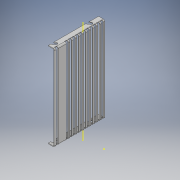
# Autodesk Inventor part: Einschub
Saved by Autodesk Inventor 2018 (Build 220112000, 112)
## iProperties
Created: 2017-11-15
Part Number: Einschub
Material: Generisch
Document SubType Name: Blech
Designer: aXe
Density: 1 g/cm^3
Sheet Metal Rule: Standard_mm
Appearance: Vorgabe
Flat Pattern Width: 14.3 cm
Flat Pattern Length: 27.2048 cm
Flat Pattern Area: 389.028 cm^2
Sheet Metal Width: 143,000 mm
Sheet Metal Length: 272,048 mm
Sheet Metal Area: 38902,834 mm^2
Author: aXe
Autodesk Inventor part; units mm, degrees
ref_plane "YZ Plane" through (0, 0, 0) normal (1, 0, 0) x (0, 1, 0)
ref_plane "XZ Plane" through (0, 0, 0) normal (0, 1, 0) x (-1, 0, 0)
ref_plane "XY Plane" through (0, 0, 0) normal (0, 0, 1) x (1, 0, 0)
ref_plane "Arbeitsebene1" through (-78, 16.4731, 8) normal (1, 0, 0) x (0, 0, 1)
sketch "Skizze1" plane through (-78, 16.4731, 8) normal (1, 0, 0) x (0, 0, 1)
  line L0 (-10, -36.2821) -> (-10, -31.9821) construction
  line L1 (-10, 63.7179) -> (-10, 68.0179) construction
  line L2 (255, 63.7179) -> (255, 68.0179) construction
  line L3 (255, -36.2821) -> (255, -31.9821) construction
  line L4 (73.6, -81.2321) -> (53.4, -81.2321) construction
  line L5 (53.4, -81.2321) -> (53.4, -79.0321) construction
  line L6 (53.4, -79.0321) -> (73.6, -79.0321) construction
  line L7 (73.6, -79.0321) -> (73.6, -81.2321) construction
  line L8 (173.4, -79.0321) -> (193.6, -79.0321) construction
  line L9 (193.6, -79.0321) -> (193.6, -81.2321) construction
  line L10 (193.6, -81.2321) -> (173.4, -81.2321) construction
  line L11 (173.4, -81.2321) -> (173.4, -79.0321) construction
  line L12 (-4, 205.8679) -> (-4, -132.095) construction
  arc A0 (-2.9629, -133.1321) -> (-4, -132.095) centre (-6.2619, -135.3941) ccw construction
  line L13 (-2.9629, -133.1321) -> (249.9629, -133.1321) construction
  arc A1 (251, -132.095) -> (249.9629, -133.1321) centre (253.2619, -135.3941) ccw construction
  line L14 (251, -132.095) -> (251, 205.8679) construction
  line L15 (226, 205.8679) -> (251, 205.8679) construction
  arc A2 (226, 205.8679) -> (221, 200.8679) centre (226, 200.8679) ccw construction
  arc A3 (216, 195.8679) -> (221, 200.8679) centre (216, 200.8679) ccw construction
  line L16 (31, 195.8679) -> (216, 195.8679) construction
  arc A4 (26, 200.8679) -> (31, 195.8679) centre (31, 200.8679) ccw construction
  arc A5 (26, 200.8679) -> (21, 205.8679) centre (21, 200.8679) ccw construction
  line L17 (-4, 205.8679) -> (21, 205.8679) construction
  line L18 (245, -237.4993) -> (245, 280.9705) construction
  line L19 (19.504, -77.1321) -> (235.504, -77.1321) construction
  line L20 (245, -237.4993) -> (245, 280.9705) construction
  line L21 (2, 280.9705) -> (2, -237.4993) construction
  line L22 (235.504, -77.1321) -> (245, -77.1321) construction
  line L23 (19.504, -77.1321) -> (2, -77.1321) construction
  line L24 (245, -77.1321) -> (245, -62.1321)
  line L25 (245, -62.1321) -> (2, -62.1321)
  line L26 (2, -62.1321) -> (2, 80.8679)
  line L27 (2, 80.8679) -> (245, 80.8679)
  line L28 (245, 80.8679) -> (245, -62.1321)
  point P0 (-8, 16.4731)
  dimension "d0" = 15
  dimension "d1" = 115
  dimension "d2" = 0
  measures "d0" distance of L22.end L24.end
  measures "d1" distance between parallel lines of L16 L27
  measures "d2" distance between parallel lines of L21 L26
extrude "Grobblech1" add sketch "Skizze1" along normal blind 2
sketch "Skizze2" plane through (-76, -64.3948, 12) normal (0, 0, -1) x (-1, 0, 0)
  line L0 (0, 143) -> (0, 0)
  line L1 (0, 0) -> (18, 0)
  line L2 (18, 0) -> (18, 143)
  line L3 (18, 143) -> (0, 143)
  constraints: 6 end point, 1 horizontal, 1 perpendicular, 1 vertical
edge flange "Lasche1" height 18 angle 90 thickness 2 bend radius 2 thickness toward (0, 0, -1) relief straight relief width 2 relief depth 1 corner gap 2 corner form 0 edges at (-78, 7.1052, 10) (-78, 7.1052, 253) wall of the first edge with corners at (-76, 78.6052, 12) (-76, -64.3948, 12) (-94, -64.3948, 12) (-94, 78.6052, 12)
bend "Biegung1"
corner "Ecke1"
sketch "Skizze3" plane through (-76, 16.4731, 8) normal (1, 0, 0) x (0, 0, -1)
  line L0 (-245, -80.8679) -> (-245, 62.1321) projected
  line L1 (-2, 62.1321) -> (-2, -80.8679) projected
  line L2 (-241, 62.1321) -> (-6, 62.1321) projected
  line L3 (-2, 62.1321) -> (-6, 62.1321) projected
  line L4 (-241, 62.1321) -> (-245, 62.1321) projected
  line L5 (-245, -80.8679) -> (-241, -80.8679) projected
  line L6 (-6, -80.8679) -> (-241, -80.8679) projected
  line L7 (-6, -80.8679) -> (-2, -80.8679) projected
  line L8 (-245, -80.8679) -> (-245, 62.1321) projected
  line L9 (-2, 62.1321) -> (-2, -80.8679) projected
  line L10 (-245, 62.1321) -> (-2, 62.1321)
  line L11 (-2, 62.1321) -> (-2, 58.1321)
  line L12 (-2, 58.1321) -> (-245, 58.1321)
  line L13 (-245, 58.1321) -> (-245, 62.1321)
  line L14 (-245, 58.1321) -> (-2, 58.1321)
  line L15 (-2, 58.1321) -> (-2, 52.1321)
  line L16 (-2, 52.1321) -> (-245, 52.1321)
  line L17 (-245, 52.1321) -> (-245, 58.1321)
  line L18 (-245, 52.1321) -> (-2, 52.1321)
  line L19 (-2, 52.1321) -> (-2, 48.1321)
  line L20 (-2, 48.1321) -> (-245, 48.1321)
  line L21 (-245, 48.1321) -> (-245, 52.1321)
  line L22 (-245, 48.1321) -> (-2, 48.1321)
  line L23 (-2, 48.1321) -> (-2, 42.1321)
  line L24 (-2, 42.1321) -> (-245, 42.1321)
  line L25 (-245, 42.1321) -> (-245, 48.1321)
  line L26 (-245, 42.1321) -> (-2, 42.1321)
  line L27 (-2, 42.1321) -> (-2, 38.1321)
  line L28 (-2, 38.1321) -> (-245, 38.1321)
  line L29 (-245, 38.1321) -> (-245, 42.1321)
  line L30 (-245, 38.1321) -> (-2, 38.1321)
  line L31 (-2, 25.9828) -> (-2, 18.6421)
  line L32 (-245, 18.6421) -> (-245, 25.9828)
  line L33 (-2, 18.6421) -> (-2, 13.3988)
  line L34 (-245, 13.3988) -> (-245, 18.6421)
  line L35 (-2, 13.3988) -> (-2, 5.0094)
  line L36 (-245, 5.0094) -> (-245, 13.3988)
  line L37 (-2, 5.0094) -> (-2, -3.5898)
  line L38 (-245, -3.5898) -> (-245, 5.0094)
  line L39 (-2, -3.5898) -> (-2, -13.2376)
  line L40 (-245, -13.2376) -> (-245, -3.5898)
  line L41 (-245, 38.1321) -> (-2, 38.1321)
  line L42 (-245, 32.1321) -> (-245, 38.1321)
  line L43 (-2, 32.1321) -> (-245, 32.1321)
  line L44 (-245, 32.1321) -> (-2, 32.1321)
  line L45 (-2, 38.1321) -> (-2, 32.1321)
  line L46 (-2, 28.1321) -> (-245, 28.1321)
  line L47 (-245, 28.1321) -> (-2, 28.1321)
  line L48 (-245, 28.1321) -> (-245, 32.1321)
  line L49 (-2, 38.1321) -> (-245, 38.1321)
  line L50 (-2, 32.1321) -> (-2, 28.1321)
  line L51 (-245, 28.1321) -> (-2, 28.1321)
  line L52 (-245, 22.1321) -> (-245, 28.1321)
  line L53 (-2, 22.1321) -> (-245, 22.1321)
  line L54 (-245, 22.1321) -> (-2, 22.1321)
  line L55 (-2, 28.1321) -> (-2, 22.1321)
  line L56 (-2, 18.1321) -> (-245, 18.1321)
  line L57 (-245, 18.1321) -> (-2, 18.1321)
  line L58 (-245, 18.1321) -> (-245, 22.1321)
  line L59 (-2, 28.1321) -> (-245, 28.1321)
  line L60 (-2, 22.1321) -> (-2, 18.1321)
  line L61 (-245, 18.1321) -> (-2, 18.1321)
  line L62 (-245, 12.1321) -> (-245, 18.1321)
  line L63 (-2, 12.1321) -> (-245, 12.1321)
  line L64 (-245, 12.1321) -> (-2, 12.1321)
  line L65 (-2, 18.1321) -> (-2, 12.1321)
  line L66 (-2, 8.1321) -> (-245, 8.1321)
  line L67 (-245, 8.1321) -> (-2, 8.1321)
  line L68 (-245, 8.1321) -> (-245, 12.1321)
  line L69 (-2, 18.1321) -> (-245, 18.1321)
  line L70 (-2, 12.1321) -> (-2, 8.1321)
  line L71 (-245, 8.1321) -> (-2, 8.1321)
  line L72 (-245, 2.1321) -> (-245, 8.1321)
  line L73 (-2, 2.1321) -> (-245, 2.1321)
  line L74 (-245, 2.1321) -> (-2, 2.1321)
  line L75 (-2, 8.1321) -> (-2, 2.1321)
  line L76 (-2, -1.8679) -> (-245, -1.8679)
  line L77 (-245, -1.8679) -> (-2, -1.8679)
  line L78 (-245, -1.8679) -> (-245, 2.1321)
  line L79 (-2, 8.1321) -> (-245, 8.1321)
  line L80 (-2, 2.1321) -> (-2, -1.8679)
  line L81 (-245, -1.8679) -> (-2, -1.8679)
  line L82 (-245, -7.8679) -> (-245, -1.8679)
  line L83 (-2, -7.8679) -> (-245, -7.8679)
  line L84 (-245, -7.8679) -> (-2, -7.8679)
  line L85 (-2, -1.8679) -> (-2, -7.8679)
  line L86 (-2, -11.8679) -> (-245, -11.8679)
  line L87 (-245, -11.8679) -> (-2, -11.8679)
  line L88 (-245, -11.8679) -> (-245, -7.8679)
  line L89 (-2, -1.8679) -> (-245, -1.8679)
  line L90 (-2, -7.8679) -> (-2, -11.8679)
  line L91 (-245, -11.8679) -> (-2, -11.8679)
  line L92 (-245, -17.8679) -> (-245, -11.8679)
  line L93 (-2, -17.8679) -> (-245, -17.8679)
  line L94 (-245, -17.8679) -> (-2, -17.8679)
  line L95 (-2, -11.8679) -> (-2, -17.8679)
  line L96 (-2, -21.8679) -> (-245, -21.8679)
  line L97 (-245, -21.8679) -> (-2, -21.8679)
  line L98 (-245, -21.8679) -> (-245, -17.8679)
  line L99 (-2, -11.8679) -> (-245, -11.8679)
  line L100 (-2, -17.8679) -> (-2, -21.8679)
  line L101 (-245, -21.8679) -> (-2, -21.8679)
  line L102 (-245, -27.8679) -> (-245, -21.8679)
  line L103 (-2, -27.8679) -> (-245, -27.8679)
  line L104 (-245, -27.8679) -> (-2, -27.8679)
  line L105 (-2, -21.8679) -> (-2, -27.8679)
  line L106 (-2, -31.8679) -> (-245, -31.8679)
  line L107 (-245, -31.8679) -> (-2, -31.8679)
  line L108 (-245, -31.8679) -> (-245, -27.8679)
  line L109 (-2, -21.8679) -> (-245, -21.8679)
  line L110 (-2, -27.8679) -> (-2, -31.8679)
  line L111 (-245, -31.8679) -> (-2, -31.8679)
  line L112 (-245, -37.8679) -> (-245, -31.8679)
  line L113 (-2, -37.8679) -> (-245, -37.8679)
  line L114 (-245, -37.8679) -> (-2, -37.8679)
  line L115 (-2, -31.8679) -> (-2, -37.8679)
  line L116 (-2, -41.8679) -> (-245, -41.8679)
  line L117 (-245, -41.8679) -> (-2, -41.8679)
  line L118 (-245, -41.8679) -> (-245, -37.8679)
  line L119 (-2, -31.8679) -> (-245, -31.8679)
  line L120 (-2, -37.8679) -> (-2, -41.8679)
  line L121 (-245, -41.8679) -> (-2, -41.8679)
  line L122 (-245, -47.8679) -> (-245, -41.8679)
  line L123 (-2, -47.8679) -> (-245, -47.8679)
  line L124 (-245, -47.8679) -> (-2, -47.8679)
  line L125 (-2, -41.8679) -> (-2, -47.8679)
  line L126 (-2, -51.8679) -> (-245, -51.8679)
  line L127 (-245, -51.8679) -> (-2, -51.8679)
  line L128 (-245, -51.8679) -> (-245, -47.8679)
  line L129 (-2, -41.8679) -> (-245, -41.8679)
  line L130 (-2, -47.8679) -> (-2, -51.8679)
  point P0 (8, -16.4731)
  dimension "d14" = 4
  dimension "d15" = 6
  dimension "d16" = 4
  dimension "d17" = 6
  dimension "d18" = 4
  dimension "d21" = 10
  constraints: 242 end point, 15 parallel, 6 horizontal, 5 perpendicular, 2 point on line, 1 vertical, 180 other
  measures "d14" distance of L10.end L11.end
  measures "d15" distance of L14.end L15.end
  measures "d16" distance of L18.end L19.end
  measures "d17" distance of L22.end L23.end
  measures "d18" distance between parallel lines of L26 L28
  measures "d21" distance of L20.end L41.start
extrude "Extrusion1" cut sketch "Skizze3" against normal blind 5 contours L0 L116 L1 L123 | L0 L106 L1 L113 | L0 L96 L1 L103 | L0 L86 L1 L93 | L0 L76 L1 L83 | L0 L66 L1 L73 | L0 L56 L1 L63 | L0 L46 L1 L53 | L0 L28 L1 L43 | L0 L20 L1 L24 | L0 L12 L1 L16
sketch "Skizze4" plane through (-76, 16.4731, 8) normal (1, 0, 0) x (0, 0, -1)
  line L0 (-243, -80.8679) -> (-245, -80.8679) projected
  line L1 (-245, -80.8679) -> (-0.3904, -80.8679)
  line L2 (-0.3904, -80.8679) -> (-0.3904, -76.8679)
  line L3 (-0.3904, -76.8679) -> (-245, -76.8679)
  line L4 (-245, -76.8679) -> (-245, -80.8679)
  line L5 (-2, -47.8679) -> (-2, -80.8679) projected
  line L6 (-245, -76.8679) -> (-2, -76.8679)
  line L7 (-2, -76.8679) -> (-2, -70.8679)
  line L8 (-2, -70.8679) -> (-245, -70.8679)
  line L9 (-245, -70.8679) -> (-245, -76.8679)
  point P0 (8, -16.4731)
  dimension "d28" = 4
  dimension "d29" = 6
  constraints: 16 end point, 4 parallel, 2 horizontal, 2 perpendicular, 1 point on line
  measures "d28" distance of L2.end L1.end
  measures "d29" distance of L7.end L6.end
extrude "Extrusion2" cut sketch "Skizze4" against normal blind 5 contours L9 L8 L5 L3
sketch "Skizze5" plane through (-94, -64.3948, 10) normal (0, 0, -1) x (-1, 0, 0)
  circle A0 centre (-6.5, 115) radius 2.15 projected
  circle A1 centre (-6.5, 15) radius 2.15 projected
  circle A2 centre (-6.5, 15) radius 4
  line L0 (0, 143) -> (0, 0) projected
  line L1 (-6.5, 15) -> (4.9414, 6.9614) construction
  line L2 (-8.7995, 11.7271) -> (2.6419, 3.6885)
  line L3 (7.2409, 10.2343) -> (-4.2005, 18.2729)
  arc A3 (-4.2005, 18.2729) -> (-8.7995, 11.7271) centre (-6.5, 15) ccw
  arc A4 (2.6419, 3.6885) -> (7.2409, 10.2343) centre (4.9414, 6.9614) ccw
  circle A5 centre (-6.5, 115) radius 4
  line L4 (-6.5, 115) -> (4.9414, 106.9614) construction
  line L5 (-8.7995, 111.7271) -> (2.6419, 103.6885)
  line L6 (7.2409, 110.2343) -> (-4.2005, 118.2729)
  arc A6 (-4.2005, 118.2729) -> (-8.7995, 111.7271) centre (-6.5, 115) ccw
  arc A7 (2.6419, 103.6885) -> (7.2409, 110.2343) centre (4.9414, 106.9614) ccw
  point P0 (-94, 64.3948)
  point P1 (-0.7793, 10.9807)
  point P2 (-0.7793, 110.9807)
  dimension "d33" = 8
  dimension "d35" = 8
  dimension "d36" = 8
  dimension "d37" = 8
  constraints: 16 end point, 8 point on circle, 8 tangent, 6 centre point, 2 midpoint, 2 parallel, 1 coincident
  measures "d33" diameter of A2
  measures "d35" diameter of A4
  measures "d36" diameter of A5
  measures "d37" diameter of A7
extrude "Extrusion3" cut sketch "Skizze5" against normal through all contours A0 | A1 | A2 | A2 L3 L0 L2 | L3 A4 L2 L0 | L6 A7 L5 L0 | L0 L5 A5 L6 | A5
sketch "Skizze6" plane through (-94, -64.3948, 12) normal (0, 0, 1) x (1, 0, 0)
  point P0 (94, 64.3948)
equation "\"d14\" = d16"
equation "\"d17\" = d15"
equation "\"d18\" = d16"
equation "\"d3\" = Stärke"
equation "\"d4\" = BreiteBiegungsfreistellung"
equation "\"d5\" = TiefeBiegungsfreistellung"
equation "\"d6\" = MinimalRest"
equation "\"d7\" = Übergangsradius"
equation "\"d10\" = Biegeradius"
equation "\"d11\" = GrößeEckenfreistellung"
equation "\"d12\" = Abstandsgröße"
equation "\"d13\" = JacobiRadiusGröße"
equation "\"Biegeradius\" = Stärke"
equation "\"BreiteBiegungsfreistellung\" = Stärke"
equation "\"TiefeBiegungsfreistellung\" = 0.5 * Stärke"
equation "\"GrößeEckenfreistellung\" = 4 * Stärke"
equation "\"MinimalRest\" = 2 * Stärke"
equation "\"Übergangsradius\" = Biegeradius"
equation "\"JacobiRadiusGröße\" = Biegeradius"
equation "\"Abstandsgröße\" = Stärke"
equation "\"Stärke\" = 2"
